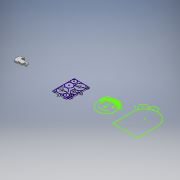
# Autodesk Inventor part: 240405_sketch
Saved by Autodesk Inventor 2016 (Build 200138000, 138)
## iProperties
Created: 2024-04-05
Part Number: 240405_sketch
Material: 일반
Document SubType Name: Modeling
Designer: pc
Density: 1 g/cm^3
Appearance: 기본값
Author: pc
Autodesk Inventor part; units mm, degrees
ref_plane "YZ Plane" through (0, 0, 0) normal (1, 0, 0) x (0, 1, 0)
ref_plane "XZ Plane" through (0, 0, 0) normal (0, 1, 0) x (-1, 0, 0)
ref_plane "XY Plane" through (0, 0, 0) normal (0, 0, 1) x (1, 0, 0)
sketch "스케치1" plane through (0, 0, 0) normal (0, 0, 1) x (1, 0, 0)
  line L0 (-43.0108, 53.8803) -> (56.9892, 53.8803)
  line L1 (56.9892, 53.8803) -> (56.9892, -86.1197)
  line L2 (56.9892, -86.1197) -> (-43.0108, -86.1197)
  line L3 (-43.0108, -86.1197) -> (-43.0108, 53.8803)
  circle A0 centre (26.9892, 23.8803) radius 30
  circle A1 centre (36.9892, -25.1095) radius 20
  circle A2 centre (46.9892, -53.3937) radius 10
  circle A3 centre (-13.0108, -56.1197) radius 30
  circle A4 centre (-26.1284, 36.998) radius 16.8824
  circle A5 centre (-19.4209, -2.9146) radius 23.5898
  circle A6 centre (29.3951, -71.1342) radius 14.9855
  circle A7 centre (49.9445, -79.0749) radius 7.0447
  arc A8 (223.6576, -12.6226) -> (232.5491, 20.6753) centre (181.7594, 16.4014) ccw
  line L4 (223.6576, -12.6226) -> (239.794, -10.976)
  arc A9 (207.192, -32.0521) -> (268.7735, -18.5502) centre (225.0108, 33.8638) ccw
  arc A10 (207.192, 11.7465) -> (186.7746, 8.1241) centre (198.9153, -0.954) ccw
  arc A11 (273.3839, 20.6753) -> (253.9544, 16.4014) centre (265.0577, 12.226) ccw
  circle A12 centre (235.1836, -2.9146) radius 59.2565
  circle A13 centre (200.6337, 45.2272) radius 8.5454
  circle A14 centre (207.9175, 49.6961) radius 8.1015
  circle A15 centre (225.0108, 53.7727) radius 9.3516
  circle A16 centre (239.6343, 51.9227) radius 11.4052
  circle A17 centre (257.9062, 45.2272) radius 9.4149
  circle A18 centre (276.3477, 45.2272) radius 10.1093
  circle A19 centre (186.7746, 35.8123) radius 9.4825
  circle A20 centre (257.9062, 60.4848) radius 8.8364
  circle A21 centre (186.7746, 55.3365) radius 12.4008
  circle A22 centre (207.9175, 60.4848) radius 9.1928
  circle A23 centre (220.0352, 67.7373) radius 6.0198
  circle A24 centre (231.7701, 67.6579) radius 7.0526
  circle A25 centre (177.2921, 23.8114) radius 9.6817
  circle A26 centre (174.3738, 42.9357) radius 7.163
  circle A27 centre (249.0698, 60.4848) radius 7.173
  circle A28 centre (268.7735, 57.7976) radius 5.7178
  circle A29 centre (241.8968, 71.3522) radius 7.0475
  circle A30 centre (288.5323, 33.493) radius 8.8105
  line L5 (356.5701, -79.6844) -> (527.6088, -79.6844)
  line L6 (527.6088, -79.6844) -> (527.6088, 51.8942)
  line L7 (356.3768, -79.6844) -> (356.3768, 51.8942)
  arc A31 (527.6088, 51.8942) -> (356.3768, 51.8942) centre (441.9928, 56.2046) ccw
  arc A32 (441.9928, 141.929) -> (393.1944, 126.6844) centre (415.4138, 141.2843) ccw
  arc A33 (392.3451, 127.2773) -> (363.8326, 94.531) centre (366.5142, 120.9822) ccw
  point P0 (335.4461, 97.2168)
  dimension "d0" = 100
  dimension "d1" = 140
  dimension "d2" = 60
  dimension "d3" = 40
  dimension "d4" = 20
  dimension "d5" = 60
  constraints: 32 centre point, 20 tangent, 18 point on circle, 16 end point, 3 horizontal, 2 parallel, 2 perpendicular, 1 horizontal alignment, 1 point on line, 1 vertical, 5 other
  measures "d0" distance of L1.end L2.end
  measures "d1" distance of L0.end L1.end
  measures "d2" diameter of A0
  measures "d3" diameter of A1
  measures "d4" diameter of A2
  measures "d5" diameter of A3
sketch "스케치2" plane through (0, 0, 0) normal (0, 0, 1) x (1, 0, 0)
  line L0 (-355.5513, -38.3336) -> (-355.5513, -14.3336)
  line L1 (-355.5513, -14.3336) -> (-345.5513, -4.3336)
  line L2 (-345.5513, -4.3336) -> (-323.5513, -4.3336)
  line L3 (-323.5513, -4.3336) -> (-323.5513, -10.3336)
  line L4 (-323.5513, -10.3336) -> (-333.5513, -10.3336)
  line L5 (-333.5513, -10.3336) -> (-333.5513, -20.3336)
  line L6 (-333.5513, -20.3336) -> (-283.5513, -20.3336)
  line L7 (-283.5513, -20.3336) -> (-277.573, -40.3336)
  line L8 (-277.573, -40.3336) -> (-287.573, -40.3336)
  line L9 (-287.573, -40.3336) -> (-287.573, -30.3336)
  line L10 (-287.573, -30.3336) -> (-297.573, -30.3336)
  line L11 (-297.573, -30.3336) -> (-297.573, -40.3336)
  line L12 (-297.573, -40.3336) -> (-299.9079, -46.7487)
  line L13 (-299.9079, -46.7487) -> (-319.9079, -46.7487)
  line L14 (-319.9079, -46.7487) -> (-319.9079, -44.7487)
  line L15 (-319.9079, -44.7487) -> (-327.2287, -44.7487)
  line L16 (-327.2287, -44.7487) -> (-327.2287, -52.7487)
  line L17 (-327.2287, -52.7487) -> (-347.2287, -52.7487)
  line L18 (-347.2287, -52.7487) -> (-355.5513, -38.3336)
  point P0 (0, 0)
  point P1 (-323.5513, -7.3336)
  dimension "d6" = 24
  dimension "d8" = 22
  dimension "d9" = 6
  dimension "d10" = 10
  dimension "d11" = 10
  dimension "d12" = 50
  dimension "d14" = 10
  dimension "d15" = 10
  dimension "d16" = 10
  dimension "d17" = 10
  dimension "d18" = 20
  dimension "d19" = 2
  dimension "d20" = 70
  dimension "d21" = 8
  dimension "d22" = 20
  dimension "d23" = 60
  dimension "d25" = 10
  dimension "d26" = 10
  dimension "d27" = 20
  constraints: 38 end point, 5 vertical, 4 horizontal, 4 perpendicular, 1 midpoint, 1 point on line
  measures "d6" distance of L0.start L0.end
  measures "d8" distance of L1.end L2.end
  measures "d9" distance of L2.end L3.end
  measures "d10" distance of L3.end L4.end
  measures "d11" distance of L4.end L5.end
  measures "d12" distance of L5.end L6.end
  measures "d14" distance of L7.end L8.end
  measures "d15" distance of L8.end L9.end
  measures "d16" distance of L9.end L10.end
  measures "d17" distance of L10.end L11.end
  measures "d18" distance of L12.end L13.end
  measures "d19" distance of L13.end L14.end
  measures "d20" angle of L13 L12
  measures "d21" distance of L15.end L16.end
  measures "d22" distance of L16.end L17.end
  measures "d23" angle of L17 L18
  measures "d25" horizontal distance of L0.end L1.end
  measures "d26" horizontal distance of L0.end L1.end
  measures "d27" distance between parallel lines of L8 L6
extrude "돌출1" add sketch "스케치2" along normal blind 10
